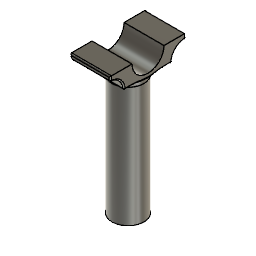
Leg (Autodesk Fusion 360 design; units mm, degrees)
Autodesk Fusion 360 part; units mm, degrees
sketch "Sketch1" plane through (0, 0, 0) normal (1, 0, 0) x (0, 1, 0)
  line L0 (0, 0) -> (0, 36.1324) construction
  line L1 (-19.05, 0) -> (19.05, 0)
  line L2 (-50, 15) -> (50, 15) construction
  arc A0 (-12.7, 15) -> (12.7, 15) centre (0, 15) ccw
  line L3 (-50, 0) -> (50, 0) construction
  arc A1 (30.05, 11) -> (19.05, 0) centre (30.05, 0) ccw
  line L4 (30.05, 0) -> (30.05, 12.671) construction
  line L5 (30.05, 11) -> (30.05, 15)
  line L6 (12.7, 15) -> (30.05, 15)
  line L7 (-12.7, 15) -> (-30.05, 15)
  line L8 (-30.05, 11) -> (-30.05, 15)
  arc A2 (-19.05, 0) -> (-30.05, 11) centre (-30.05, 0) ccw
  point P0 (0, 15)
  dimension "d2" = 38.1
  dimension "d3" = 100
  dimension "d4" = 12.7
  dimension "d5" = 100
  dimension "d6" = 15
  dimension "d7" = 4
  constraint coincident L0.start origin
  constraint midpoint L1 L0.start
  constraint horizontal L1
  constraint midpoint L2 P0
  constraint perpendicular L0 L2
  constraint coincident L2 A0.start
  constraint coincident L2 A0.end
  constraint coincident L2 P0
  constraint coincident L0 P0
  constraint vertical L0
  constraint coincident P0 A0.centre
  constraint midpoint L3 L0.start
  constraint perpendicular L0 L3
  constraint coincident L3 A1.centre
  constraint coincident A1.centre L4.start
  constraint perpendicular L3 L4
  constraint coincident A1.start L4
  constraint coincident L2 L5.end
  constraint perpendicular L2 L5
  constraint symmetric L0 L1.end L1.start
  constraint symmetric L0 A0.end A0.start
  constraint symmetric L0 A1.start L8.start
  constraint symmetric L0 A1 A2
  constraint symmetric L0 L5.end L7.end
  measures "d2" distance of L1.start L1.end
  measures "d3" distance of L2.start L2.end
  measures "d4" radius of A0
  measures "d5" distance of L3.start L3.end
  measures "d6" distance of L2 L3
  measures "d7" distance of L2 A1.start
extrude "Extrude1" add sketch "Sketch1" along normal mid plane 31.75
sketch "Sketch2" plane through (0, 0, 0) normal (0, 0, -1) x (1, 0, 0)
  line L0 (-15.875, -19.05) -> (15.875, -19.05)
  line L1 (15.875, -19.05) -> (15.875, 19.05)
  line L2 (15.875, 19.05) -> (-15.875, 19.05)
  line L3 (-15.875, 19.05) -> (-15.875, -19.05)
  circle A0 centre (0, 0) radius 12.7
  circle A1 centre (0, 0) radius 8.7
  dimension "d10" = 25.4
  dimension "d11" = -4
  constraint coincident A0.centre A1.centre
  measures "d10" diameter of A0
extrude "Extrude2" add sketch "Sketch2" along normal blind 101.6 contours A0
fillet "Fillet1" radius 6.35 1 edges at (-11.8406, -4.5925, 0)
fillet "Fillet2" radius 2 1 edges at (-15.875, -22.2718, 7.7782)
fillet "Fillet2" radius 1 21 edges at (0, -30.05, 11) (15.875, -22.2718, 7.7782) (-7.9375, -19.05, 0) (7.9375, -19.05, 0) (0, -30.05, 15) (15.875, -14.7901, 0) (15.875, 0, -0.8507) (15.875, 14.7901, 0) (-15.875, 14.7901, 0) (-15.875, 0, -0.8507) (-15.875, -14.7901, 0) (-7.9375, 19.05, 0) (7.9375, 19.05, 0) (-15.875, 22.2718, 7.7782) (0, 30.05, 11) (15.875, 22.2718, 7.7782) (0, 30.05, 15) (15.875, 30.05, 13) (15.875, -30.05, 13) (-15.875, -30.05, 13) (-15.875, 30.05, 13)
equation "d4 = 1 in / 2"
